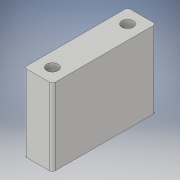
# Autodesk Inventor part: Bearing Seats
Saved by Autodesk Inventor 2019 (Build 230136000, 136)
## iProperties
Created: 2019-11-26
Part Number: Bearing Seats
Material: Generic
Document SubType Name: Modeling
Designer: micha
Density: 1 g/cm^3
Appearance: Default
Author: micha
Autodesk Inventor part; units mm, degrees
ref_plane "YZ Plane" through (0, 0, 0) normal (1, 0, 0) x (0, 1, 0)
ref_plane "XZ Plane" through (0, 0, 0) normal (0, 1, 0) x (-1, 0, 0)
ref_plane "XY Plane" through (0, 0, 0) normal (0, 0, 1) x (1, 0, 0)
sketch "Sketch1" plane through (0, 0, 0) normal (0, 1, 0) x (-1, 0, 0)
  line L0 (0, 0) -> (0, -53)
  circle A0 centre (0, 0) radius 4
  circle A1 centre (0, -53) radius 4
  line L1 (0, 10) -> (10, 10)
  line L2 (0, -63) -> (-10, -63)
  line L3 (10, 10) -> (-10, 10)
  line L4 (-10, 10) -> (-10, -63)
  line L5 (-10, -63) -> (10, -63)
  line L6 (10, -63) -> (10, 10)
  dimension "d0" = 53
  dimension "d1" = 8
  dimension "d2" = 8
  dimension "d3" = 10
  dimension "d4" = 10
  dimension "d5" = 10
  dimension "d6" = 10
  dimension "d8" = 10
  dimension "d9" = 10
  dimension "d10" = 73
  constraints: 14 end point, 2 centre point, 2 coincident, 2 parallel, 1 horizontal, 1 perpendicular, 1 vertical
  measures "d0" distance of L0.start L0.end
  measures "d1" diameter of A0
  measures "d2" diameter of A1
  measures "d3" distance of A0.centre L1.start
  measures "d4" distance of L1.start L1.end
  measures "d5" distance of A1.centre L2.start
  measures "d6" distance of L2.start L2.end
  measures "d8" distance between parallel lines of L6 L0
  measures "d9" distance between parallel lines of L4 L0
  measures "d10" distance between parallel lines of L1 L5
extrude "Extrusion1" add sketch "Sketch1" along normal blind 54
fillet "Fillet1" radius 2 4 edges at (10, 27, 10) (-10, 27, 10) (10, 27, -63) (-10, 27, -63)
body "Solid1"
